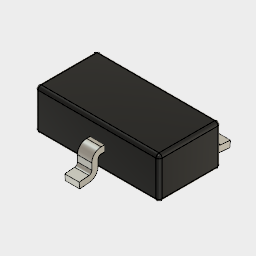
SOP-3 (Autodesk Fusion 360 design; units mm, degrees)
Autodesk Fusion 360 part; units mm, degrees
ref_plane "WorkPlane1" through (0, 0, 0.05) normal (0, 0, 1) x (1, 0, 0)
sketch "Sketch1" plane through (0, 0, 0.05) normal (0, 0, 1) x (1, 0, 0)
  line L0 (1.5, 0.75) -> (-1.5, 0.75)
  line L1 (-1.5, 0.75) -> (-1.5, -0.75)
  line L2 (-1.5, -0.75) -> (1.5, -0.75)
  line L3 (1.5, -0.75) -> (1.5, 0.75)
  line L4 (1.5, 0.75) -> (-1.5, -0.75) construction
  line L5 (-1.5, 0.75) -> (1.5, -0.75) construction
  dimension "d2" = 3
  dimension "d3" = 1.5
  measures "d2" distance of L1.end L2.end
  measures "d3" distance of L0.end L1.end
extrude "Extrude1" add sketch "Sketch1" along normal blind 1 makes body 1
sketch "Sketch2" plane through (0, -0.75, 0) normal (0, -1, 0) x (1, 0, 0)
  line L0 (-1.5, 0.05) -> (1.5, 0.05)
  line L1 (1.5, 0.05) -> (1.5, 1.05)
  line L2 (1.5, 1.05) -> (-1.5, 1.05)
  line L3 (-1.5, 1.05) -> (-1.5, 0.05)
  line L4 (0.175, 0.475) -> (-0.175, 0.475)
  line L5 (-0.175, 0.475) -> (-0.175, 0.625)
  line L6 (-0.175, 0.625) -> (0.175, 0.625)
  line L7 (0.175, 0.625) -> (0.175, 0.475)
  line L8 (0.175, 0.475) -> (-0.175, 0.625) construction
  line L9 (-0.175, 0.475) -> (0.175, 0.625) construction
  point P0 (0, 0.55)
  dimension "d6" = 0.35
  dimension "d7" = 0.15
  dimension "d8" = 0.5
  measures "d6" distance of L5.end L6.end
  measures "d7" distance of L4.end L5.end
  measures "d8" distance of L0 P0
sketch "Sketch3" plane through (0, 0, 0) normal (1, 0, 0) x (0, 1, 0)
  line L0 (-0.75, 0.55) -> (-0.825, 0.55)
  arc A0 (-0.825, 0.55) -> (-0.975, 0.4) centre (-0.825, 0.4) ccw
  line L1 (-0.975, 0.4) -> (-0.975, 0.2453)
  arc A1 (-1.1119, 0.0958) -> (-0.975, 0.2453) centre (-1.125, 0.2453) ccw
  line L2 (-1.1119, 0.0958) -> (-1.35, 0.075)
  line L3 (-0.75, 0.625) -> (-0.75, 0.475)
  line L4 (-0.75, 0.55) -> (-0.6, 0.55)
  line L5 (-1.35, 0.075) -> (-0.85, 0.075) construction
  point P0 (-0.75, 0.55)
  dimension "d10" = 0.15
  dimension "d11" = 0.075
  dimension "d21" = 0.15
  dimension "d22" = 0.225
  dimension "d23" = 0.6
  dimension "d24" = 0.5
  dimension "d25" = 5
  dimension "d26" = 0.15
  measures "d10" radius of A0
  measures "d11" distance of origin L2.end
  measures "d21" distance of P0 L4.end
  measures "d22" distance of P0 L1
  measures "d23" distance of P0 L2.end
  measures "d24" distance of L2.end L5.end
  measures "d25" angle of L2 L5
  measures "d26" radius of A1
sweep "Sweep1" add profiles "Sketch2" path "Sketch3" along L2 A1 L1 A0 L0 L4 section 1 contours L4 L5 L6 L7 separate body makes body 2
pattern_linear "R-Pattern1" count 3 spacing 0.95 along (1, 0, 0) both ways of "Sweep1" makes body 3 makes body 4
fillet "Fillet1" radius 0.075 12 edges at (1.5, 0, 1.05) (0, -0.75, 1.05) (-1.5, 0, 1.05) (0, 0.75, 1.05) (1.5, -0.75, 0.55) (1.5, 0, 0.05) (1.5, 0.75, 0.55) (0, -0.75, 0.05) (-1.5, -0.75, 0.55) (-1.5, 0, 0.05) (0, 0.75, 0.05) (-1.5, 0.75, 0.55) on bodies 1
move_body "Move1" bodies 3 4 to x (-1, 0, 0) y (0, -1, 0) z (0, 0, 1) at (0, 0, 0)
equation "d1 = sop3_above_board"
equation "d2 = sop3_package_width"
equation "d3 = sop3_package_depth"
equation "d4 = sop3_package_height"
equation "d6 = sop3_lead_width"
equation "d7 = sop3_lead_thickness"
equation "d8 = sop3_lead_attach"
equation "d10 = sop3_lead_thickness"
equation "d11 = sop3_lead_thickness / 2"
equation "sop3_lead_thickness = 0.15 mm"
equation "sop3_lead_attach = 0.5 mm"
equation "sop3_lead_width = 0.35 mm"
equation "sop3_lead_spacing = 0.95 mm"
equation "sop3_package_width = 3 mm"
equation "sop3_package_height = 1 mm"
equation "sop3_package_depth = 1.5 mm"
equation "sop3_above_board = 0.05 mm"
equation "d21 = sop3_lead_into_package"
equation "d22 = sop3_lead_thickness * ( 3 / 2 )"
equation "d23 = sop3_lead_extension"
equation "d25 = sop3_lead_foot_angle"
equation "d26 = d10"
equation "sop3_lead_extension = 0.6 mm"
equation "sop3_lead_foot_angle = 5 deg"
equation "sop3_lead_into_package = 0.15 mm"
equation "d34 = sop3_lead_spacing"
equation "sop3_optional_lead_extension = 0 mm"
named bodies: "lead2", "lead1", "lead3"
